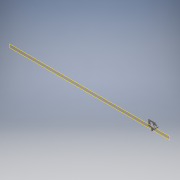
# Autodesk Inventor part: YMotorMount
Saved by Autodesk Inventor 2016 (Build 200138000, 138)
## iProperties
Created: 2016-05-31
Part Number: YMotorMount
Material: Generic
Document SubType Name: Modeling
Designer: Scott
Density: 1 g/cm^3
Appearance: Default
Author: Scott
Autodesk Inventor part; units mm, degrees
ref_plane "YZ Plane" through (0, 0, 0) normal (1, 0, 0) x (0, 1, 0)
ref_plane "XZ Plane" through (0, 0, 0) normal (0, 1, 0) x (-1, 0, 0)
ref_plane "XY Plane" through (0, 0, 0) normal (0, 0, 1) x (1, 0, 0)
ref_plane "Work Plane1" through (0, 0, 0) normal (0, 0, 1) x (1, 0, 0)
sketch "Sketch1" plane through (0, 0, 0) normal (0, 0, 1) x (1, 0, 0)
  line L0 (374.65, 19.755) -> (374.65, -0.245) projected
  line L1 (394.65, -0.245) -> (394.65, 19.755) projected
  line L2 (374.65, -0.245) -> (394.65, -0.245) projected
  line L3 (374.65, -0.245) -> (372.11, -0.245)
  line L4 (372.11, -0.245) -> (372.11, 19.755)
  line L5 (372.11, 19.755) -> (374.65, 19.755)
  line L6 (374.65, 19.755) -> (374.65, -0.245)
  line L7 (372.11, 19.755) -> (394.65, 19.755)
  line L8 (394.65, 19.755) -> (394.65, 24.835)
  line L9 (394.65, 24.835) -> (372.11, 24.835)
  line L10 (372.11, 24.835) -> (372.11, 19.755)
  point P0 (0, 0)
  dimension "d0" = 2.54
  dimension "d1" = 20
  dimension "d2" = 5.08
  constraints: 16 end point, 4 parallel, 2 horizontal, 2 perpendicular
  measures "d0" distance of L4.end L5.end
  measures "d1" distance of L3.end L4.end
  measures "d2" distance of L8.end L7.end
extrude "Extrusion1" add sketch "Sketch1" along normal mid plane 20 contours L0 L3 L4 L5 | L5 L10 L9 L8 L7
sketch "Sketch2" plane through (372.11, 24.835, -10) normal (0, 1, 0) x (1, 0, 0)
  line L0 (0, 0) -> (22.54, 0) projected
  line L1 (0, 0) -> (0, -20) projected
  line L2 (22.54, -20) -> (0, -20) projected
  line L3 (22.54, 0) -> (22.54, -20) projected
  line L4 (2.54, -340.2) -> (2.54, 320.2) projected
  line L5 (2.54, -20) -> (2.54, 0) projected
  line L6 (2.54, -10) -> (22.54, -10)
  circle A0 centre (12.54, -10) radius 2.5
  point P0 (-372.11, -10)
  dimension "d5" = 5
  constraints: 3 midpoint, 2 end point, 1 centre point
  measures "d5" diameter of A0
extrude "Extrusion2" cut sketch "Sketch2" against normal blind 20 contours A0 L6 | L6 A0
sketch "Sketch3" plane through (374.65, -0.245, -10) normal (1, 0, 0) x (0, 0, -1)
  line L0 (0, 20) -> (0, 0) projected
  line L1 (0, 20) -> (-20, 20) projected
  circle A0 centre (-10, 10) radius 2.5
  point P0 (-10, 0.245)
  dimension "d8" = 5
  constraints: 1 centre point, 1 other
  measures "d8" diameter of A0
extrude "Extrusion3" cut sketch "Sketch3" against normal blind 20
sketch "Sketch4" plane through (0, 0, -10) normal (0, 0, -1) x (-1, 0, 0)
  line L0 (-374.65, -0.245) -> (-374.65, 19.755) projected
  line L1 (-374.65, 19.755) -> (-394.65, 19.755) projected
  line L2 (-394.65, 19.755) -> (-394.65, 24.835) projected
  line L3 (-394.65, 24.835) -> (-372.11, 24.835) projected
  line L4 (-372.11, 24.835) -> (-372.11, -0.245) projected
  line L5 (-372.11, -0.245) -> (-374.65, -0.245) projected
  line L6 (-372.11, -0.245) -> (-330.11, -0.245)
  line L7 (-330.11, -0.245) -> (-330.11, 41.755)
  line L8 (-330.11, 41.755) -> (-372.11, 41.755)
  line L9 (-372.11, 41.755) -> (-372.11, -0.245)
  circle A0 centre (-351.11, 20.755) radius 12.5
  circle A1 centre (-335.61, 36.255) radius 2
  circle A2 centre (-335.61, 5.255) radius 2
  circle A3 centre (-366.61, 36.255) radius 2
  circle A4 centre (-366.61, 5.255) radius 2
  point P0 (0, 0)
  dimension "d11" = 42
  dimension "d12" = 42
  dimension "d13" = 25
  dimension "d16" = 4
  dimension "d19" = 31
  dimension "d22" = 31
  constraints: 8 end point, 5 centre point, 2 horizontal, 2 parallel, 1 perpendicular, 1 vertical, 6 other
  measures "d11" distance of L8.end L7.end
  measures "d12" distance of L7.end L6.end
  measures "d13" diameter of A0
  measures "d16" diameter of A1
  measures "d19" distance of A1.centre A2.centre
  measures "d22" distance of A1.centre A3.centre
extrude "Extrusion4" add sketch "Sketch4" along normal blind 5.08
chamfer "Chamfer1" distance 16.764 angle 45 1 edges at (372.11, 24.835, -12.54)
body "Solid1"
